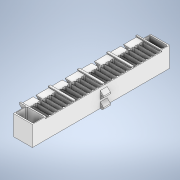
# Autodesk Inventor part: cajas_V2
Saved by Autodesk Inventor 2020.3 (Build 243373000, 373)
## iProperties
Created: 2021-02-18
Part Number: cajas_V2
Material: PET Plastic
Document SubType Name: Modeling
Designer: juanp
Density: 1.541 g/cm^3
Appearance: Polycarbonate - Clear
Author: juanp
Autodesk Inventor part; units mm, degrees
ref_plane "YZ Plane" through (0, 0, 0) normal (1, 0, 0) x (0, 1, 0)
ref_plane "XZ Plane" through (0, 0, 0) normal (0, 1, 0) x (-1, 0, 0)
ref_plane "XY Plane" through (0, 0, 0) normal (0, 0, 1) x (1, 0, 0)
sketch "Sketch1" plane through (0, 0, 0) normal (0, 1, 0) x (-1, 0, 0)
  line L0 (0, 0) -> (54, 0) construction
  line L1 (54, 0) -> (54, -330)
  line L2 (0, -330) -> (0, 0)
  line L3 (52, -4) -> (2, -4) construction
  line L4 (2, -4) -> (2, -15.1667)
  line L5 (2, -15.1667) -> (52, -15.1667)
  line L6 (52, -15.1667) -> (52, -4)
  line L7 (52, -19.1667) -> (2, -19.1667)
  line L8 (2, -19.1667) -> (2, -30.3333)
  line L9 (2, -30.3333) -> (52, -30.3333)
  line L10 (52, -30.3333) -> (52, -19.1667)
  line L11 (52, -32.3333) -> (2, -32.3333)
  line L12 (2, -32.3333) -> (2, -43.5)
  line L13 (2, -43.5) -> (52, -43.5)
  line L14 (52, -43.5) -> (52, -32.3333)
  line L15 (52, -45.5) -> (2, -45.5)
  line L16 (2, -45.5) -> (2, -56.6667)
  line L17 (2, -56.6667) -> (52, -56.6667)
  line L18 (52, -56.6667) -> (52, -45.5)
  line L19 (52, -58.6667) -> (2, -58.6667)
  line L20 (2, -58.6667) -> (2, -69.8333)
  line L21 (2, -69.8333) -> (52, -69.8333)
  line L22 (52, -69.8333) -> (52, -58.6667)
  line L23 (52, -71.8333) -> (2, -71.8333)
  line L24 (2, -71.8333) -> (2, -83)
  line L25 (2, -83) -> (52, -83)
  line L26 (52, -83) -> (52, -71.8333)
  line L27 (52, -85) -> (2, -85)
  line L28 (2, -85) -> (2, -96.1667)
  line L29 (2, -96.1667) -> (52, -96.1667)
  line L30 (52, -96.1667) -> (52, -85)
  line L31 (52, -102.1667) -> (2, -102.1667)
  line L32 (2, -102.1667) -> (2, -113.3333)
  line L33 (2, -113.3333) -> (52, -113.3333)
  line L34 (52, -113.3333) -> (52, -102.1667)
  line L35 (52, -115.3333) -> (2, -115.3333)
  line L36 (2, -115.3333) -> (2, -126.5)
  line L37 (2, -126.5) -> (52, -126.5)
  line L38 (52, -126.5) -> (52, -115.3333)
  line L39 (52, -128.5) -> (2, -128.5)
  line L40 (2, -128.5) -> (2, -139.6667)
  line L41 (2, -139.6667) -> (52, -139.6667)
  line L42 (52, -139.6667) -> (52, -128.5)
  line L43 (52, -141.6667) -> (2, -141.6667)
  line L44 (2, -141.6667) -> (2, -152.8333)
  line L45 (2, -152.8333) -> (52, -152.8333)
  line L46 (52, -152.8333) -> (52, -141.6667)
  line L47 (52, -154.8333) -> (2, -154.8333)
  line L48 (2, -154.8333) -> (2, -166)
  line L49 (2, -166) -> (52, -166)
  line L50 (52, -166) -> (52, -154.8333)
  line L51 (52, -168) -> (2, -168)
  line L52 (2, -168) -> (2, -179.1667)
  line L53 (2, -179.1667) -> (52, -179.1667)
  line L54 (52, -179.1667) -> (52, -168)
  line L55 (52, -185.1667) -> (2, -185.1667)
  line L56 (2, -185.1667) -> (2, -196.3333)
  line L57 (2, -196.3333) -> (52, -196.3333)
  line L58 (52, -196.3333) -> (52, -185.1667)
  line L59 (52, -198.3333) -> (2, -198.3333)
  line L60 (2, -198.3333) -> (2, -209.5)
  line L61 (2, -209.5) -> (52, -209.5)
  line L62 (52, -209.5) -> (52, -198.3333)
  line L63 (52, -211.5) -> (2, -211.5)
  line L64 (2, -211.5) -> (2, -222.6667)
  line L65 (2, -222.6667) -> (52, -222.6667)
  line L66 (52, -222.6667) -> (52, -211.5)
  line L67 (52, -224.6667) -> (2, -224.6667)
  line L68 (2, -224.6667) -> (2, -235.8333)
  line L69 (2, -235.8333) -> (52, -235.8333)
  line L70 (52, -235.8333) -> (52, -224.6667)
  line L71 (54, -330) -> (54, -349.1667)
  line L72 (54, -349.1667) -> (0, -349.1667) construction
  line L73 (0, -349.1667) -> (0, -330)
  line L74 (52, -237.8333) -> (2, -237.8333)
  line L75 (2, -237.8333) -> (2, -249)
  line L76 (2, -249) -> (52, -249)
  line L77 (52, -249) -> (52, -237.8333)
  line L78 (52, -251) -> (2, -251)
  line L79 (2, -251) -> (2, -262.1667)
  line L80 (2, -262.1667) -> (52, -262.1667)
  line L81 (52, -262.1667) -> (52, -251)
  line L82 (52, -268.1667) -> (2, -268.1667)
  line L83 (2, -268.1667) -> (2, -279.3333)
  line L84 (2, -279.3333) -> (52, -279.3333)
  line L85 (52, -279.3333) -> (52, -268.1667)
  line L86 (52, -281.3333) -> (2, -281.3333)
  line L87 (2, -281.3333) -> (2, -292.5)
  line L88 (2, -292.5) -> (52, -292.5)
  line L89 (52, -292.5) -> (52, -281.3333)
  line L90 (52, -294.5) -> (2, -294.5)
  line L91 (2, -294.5) -> (2, -305.6667)
  line L92 (2, -305.6667) -> (52, -305.6667)
  line L93 (52, -305.6667) -> (52, -294.5)
  line L94 (52, -307.6667) -> (2, -307.6667)
  line L95 (2, -307.6667) -> (2, -318.8333)
  line L96 (2, -318.8333) -> (52, -318.8333)
  line L97 (52, -318.8333) -> (52, -307.6667)
  line L98 (52, -320.8333) -> (2, -320.8333)
  line L99 (2, -320.8333) -> (2, -332)
  line L100 (2, -332) -> (52, -332)
  line L101 (52, -332) -> (52, -320.8333)
  line L102 (52, -334) -> (2, -334)
  line L103 (2, -334) -> (2, -345.1667)
  line L104 (2, -345.1667) -> (52, -345.1667)
  line L105 (52, -345.1667) -> (52, -334)
  line L106 (52, -4) -> (52, 16.4167)
  line L107 (52, 16.4167) -> (2, 16.4167)
  line L108 (2, 16.4167) -> (2, -4)
  line L109 (54, 0) -> (54, 20.4167)
  line L110 (54, 20.4167) -> (0, 20.4167)
  line L111 (0, 20.4167) -> (0, 0)
  line L112 (0, -349.1667) -> (0, -369.5833)
  line L113 (0, -369.5833) -> (54, -369.5833)
  line L114 (54, -369.5833) -> (54, -349.1667)
  line L115 (52, -339.5833) -> (104.9487, -339.5833) construction
  line L116 (104.9487, -339.5833) -> (104.9487, -9.5833) construction
  line L117 (104.9487, -9.5833) -> (52, -9.5833) construction
  line L118 (2, -349.1667) -> (52, -349.1667)
  line L119 (52, -349.1667) -> (52, -365.5833)
  line L120 (52, -365.5833) -> (2, -365.5833)
  line L121 (2, -365.5833) -> (2, -349.1667)
  point P0 (104.9487, -174.5833)
  dimension "d2" = 2
  dimension "d3" = 4
  dimension "d4" = 2
  dimension "d5" = 50
  dimension "d6" = 4
  dimension "d7" = 2
  dimension "d8" = 2
  dimension "d9" = 2
  dimension "d10" = 2
  dimension "d11" = 2
  dimension "d12" = 6
  dimension "d13" = 2
  dimension "d14" = 2
  dimension "d15" = 2
  dimension "d16" = 2
  dimension "d17" = 2
  dimension "d18" = 6
  dimension "d19" = 2
  dimension "d20" = 2
  dimension "d21" = 2
  dimension "d24" = 11.1667
  dimension "d35" = 2
  dimension "d36" = 2
  dimension "d37" = 6
  dimension "d38" = 2
  dimension "d39" = 2
  dimension "d40" = 2
  dimension "d41" = 2
  dimension "d42" = 2
  dimension "d59" = 4
  dimension "d60" = 330
  dimension "d212" = 4
  dimension "d332" = 195
  dimension "d333" = 195
  dimension "d334" = 4
  constraints: 244 end point, 53 parallel, 37 perpendicular, 34 equal length, 33 point on line, 28 horizontal, 8 collinear, 5 vertical, 3 midpoint
  measures "d2" distance between parallel lines of L1 L6
  measures "d3" distance between parallel lines of L0 L3
  measures "d4" distance between parallel lines of L4 L2
  measures "d5" distance of L3.start L3.end
  measures "d6" distance between parallel lines of L7 L5
  measures "d7" distance between parallel lines of L11 L9
  measures "d8" distance between parallel lines of L15 L13
  measures "d9" distance between parallel lines of L19 L17
  measures "d10" distance between parallel lines of L21 L23
  measures "d11" distance between parallel lines of L27 L25
  measures "d12" distance between parallel lines of L31 L29
  measures "d13" distance between parallel lines of L35 L33
  measures "d14" distance between parallel lines of L39 L37
  measures "d15" distance between parallel lines of L43 L41
  measures "d16" distance between parallel lines of L47 L45
  measures "d17" distance between parallel lines of L51 L49
  measures "d18" distance between parallel lines of L55 L53
  measures "d19" distance between parallel lines of L59 L57
  measures "d20" distance between parallel lines of L63 L61
  measures "d21" distance between parallel lines of L67 L65
  measures "d24" distance of L61.end L59.start
  measures "d35" distance between parallel lines of L69 L74
  measures "d36" distance between parallel lines of L78 L76
  measures "d37" distance between parallel lines of L82 L80
  measures "d38" distance between parallel lines of L86 L84
  measures "d39" distance between parallel lines of L90 L88
  measures "d40" distance between parallel lines of L94 L92
  measures "d41" distance between parallel lines of L98 L96
  measures "d42" distance between parallel lines of L102 L100
  measures "d59" distance between parallel lines of L72 L104
  measures "d60" distance of L117.end L115.start
  measures "d212" distance between parallel lines of L107 L110
  measures "d332" distance from line of L110 point (104.949, -174.583)
  measures "d333" distance from line of L113 point (104.949, -174.583)
  measures "d334" distance between parallel lines of L113 L120
extrude "Extrusion1" add sketch "Sketch1" along normal blind 50
sketch "Sketch3" plane through (0, 0, 0) normal (0, -1, 0) x (1, 0, 0)
  line L0 (-54, -369.5833) -> (-54, 20.4167) projected
  line L1 (0, 20.4167) -> (0, -369.5833) projected
  line L2 (-54, 20.4167) -> (0, 20.4167) projected
  line L3 (0, -369.5833) -> (-54, -369.5833) projected
extrude "Extrusion3" add sketch "Sketch3" along normal blind 2
chamfer "Chamfer4" distance 2 angle 45 208 edges at (-52, 25, -128.5) (-2, 25, -126.5) (-52, 25, -141.6667) (-52, 25, -179.1667) (-52, 25, -185.1667) (-2, 25, -141.6667) (-2, 25, -139.6667) (-52, 25, -115.3333) (-2, 25, -115.3333) (-2, 25, -345.1667) (-52, 25, -345.1667) (-2, 25, -128.5) (-2, 25, -332) (-2, 25, -334) (-52, 25, -334) (-52, 25, -332) (-2, 25, -320.8333) (-52, 25, -318.8333) (-2, 25, -318.8333) (-52, 25, -320.8333) (-2, 25, -307.6667) (-52, 25, -305.6667) (-52, 25, -307.6667) (-2, 25, -305.6667) (-2, 25, -294.5) (-52, 25, -292.5) (-2, 25, -292.5) (-52, 25, -294.5) (-2, 25, -281.3333) (-2, 25, -268.1667) (-52, 25, -279.3333) (-2, 25, -279.3333) (-52, 25, -281.3333) (-2, 25, -166) (-2, 25, -168) (-2, 25, -179.1667) (-2, 25, -196.3333) (-2, 25, -185.1667) (-2, 25, -209.5) (-2, 25, -198.3333) (-52, 0, -173.5833) (-2, 0, -173.5833) (-27, 0, -179.1667) (-27, 0, -185.1667) (-52, 0, -190.75) (-2, 0, -190.75) (-2, 0, -203.9167) (-27, 0, -198.3333) (-52, 0, -203.9167) (-27, 0, -196.3333) (-52, 0, -217.0833) (-2, 0, -217.0833) (-27, 0, -222.6667) (-27, 0, -209.5) (-52, 25, -196.3333) (-52, 25, -198.3333) (-52, 25, -209.5) (-2, 25, -211.5) (-52, 25, -211.5) (-52, 25, -222.6667) (-2, 25, -222.6667) (-2, 25, -224.6667) (-52, 25, -224.6667) (-2, 25, -251) (-52, 25, -249) (-2, 25, -249) (-52, 25, -251) (-2, 25, -262.1667) (-52, 25, -262.1667) (-52, 25, -268.1667) (-27, 0, -211.5) (-27, 0, -224.6667) (-52, 0, -230.25) (-2, 0, -230.25) (-27, 0, -235.8333) (-27, 0, -237.8333) (-52, 0, -243.4167) (-2, 0, -243.4167) (-27, 0, -249) (-27, 0, -251) (-52, 0, -256.5833) (-27, 0, -262.1667) (-27, 0, -268.1667) (-52, 0, -273.75) (-27, 0, -279.3333) (-2, 0, -273.75) (-52, 0, -286.9167) (-27, 0, -292.5) (-2, 0, -256.5833) (-27, 0, -281.3333) (-2, 0, -286.9167) (-27, 0, -294.5) (-52, 0, -300.0833) (-2, 0, -300.0833) (-27, 0, -305.6667) (-27, 0, -307.6667) (-52, 0, -313.25) (-2, 0, -313.25) (-27, 0, -318.8333) (-27, 0, -320.8333) (-27, 0, -332) (-2, 0, -326.4167) (-27, 0, -334) (-2, 0, -339.5833) (-27, 0, -345.1667) (-52, 0, -339.5833) (-52, 0, -326.4167) (-2, 25, -237.8333) (-2, 25, -235.8333) (-52, 25, -235.8333) (-52, 25, -237.8333) (-52, 25, -126.5) (-52, 25, -113.3333) (-2, 25, -113.3333) (-2, 25, -102.1667) (-52, 25, -102.1667) (-52, 25, -96.1667) (-2, 25, -96.1667) (-2, 25, -85) (-52, 25, -85) (-27, 0, -96.1667) (-2, 0, -90.5833) (-27, 0, -85) (-27, 0, -83) (-2, 0, -77.4167) (-27, 0, -71.8333) (-52, 0, -77.4167) (-52, 0, -90.5833) (-52, 25, -83) (-2, 25, -83) (-2, 25, -71.8333) (-52, 25, -71.8333) (-52, 25, -69.8333) (-2, 25, -69.8333) (-2, 25, -58.6667) (-52, 25, -58.6667) (-52, 25, -56.6667) (-52, 25, -45.5) (-52, 25, -43.5) (-2, 25, -56.6667) (-52, 25, -32.3333) (-2, 25, -43.5) (-52, 25, -30.3333) (-2, 25, -32.3333) (-2, 25, -30.3333) (-52, 25, -19.1667) (-2, 25, -19.1667) (-2, 25, -45.5) (-52, 0, -24.75) (-52, 25, -15.1667) (-2, 25, -15.1667) (-27, 0, -43.5) (-27, 0, -32.3333) (-2, 0, -37.9167) (-27, 0, -30.3333) (-2, 0, -24.75) (-27, 0, -19.1667) (-52, 0, -37.9167) (-27, 0, -69.8333) (-52, 0, -64.25) (-2, 0, -64.25) (-27, 0, -58.6667) (-27, 0, -56.6667) (-2, 0, -51.0833) (-27, 0, -45.5) (-52, 0, -51.0833) (-2, 25, -154.8333) (-2, 25, -152.8333) (-52, 25, -152.8333) (-52, 25, -139.6667) (-27, 0, -168) (-27, 0, -166) (-27, 0, -154.8333) (-2, 0, -160.4167) (-27, 0, -152.8333) (-2, 0, -147.25) (-27, 0, -141.6667) (-2, 0, -134.0833) (-27, 0, -128.5) (-52, 0, -147.25) (-52, 0, -160.4167) (-27, 0, -102.1667) (-52, 0, -107.75) (-2, 0, -107.75) (-27, 0, -113.3333) (-27, 0, -115.3333) (-27, 0, -126.5) (-2, 0, -120.9167) (-27, 0, -139.6667) (-52, 0, -134.0833) (-52, 0, -120.9167) (-52, 25, -154.8333) (-52, 25, -166) (-52, 25, -168) (-2, 25, 16.4167) (-52, 25, 16.4167) (-27, 0, 16.4167) (-52, 0, 0.625) (-27, 0, -15.1667) (-2, 0, 0.625) (-27, 0, -365.5833) (-2, 0, -357.375) (-2, 25, -365.5833) (-52, 25, -349.1667) (-52, 0, -357.375) (-27, 0, -349.1667) (-2, 25, -349.1667) (-52, 25, -365.5833)
ref_plane "Plano medio efectivo" through (-4, 2, -174.5833) normal (0, 0, -1) x (-1, 0, 0)
sketch "Sketch57" plane through (-4, 50, -349.1667) normal (0, 0, -1) x (-1, 0, 0)
  line L0 (50, -52) -> (50, 0) projected
  line L1 (50, 0) -> (67.933, 0)
  line L2 (67.933, 0) -> (50, -17.933)
  point P0 (-4, -50)
  dimension "d335" = 45
  dimension "d336" = 17.933
  constraints: 4 end point, 1 horizontal, 1 point on line
  measures "d335" angle of L0 L2
  measures "d336" distance of L0.end L1.end
extrude "Extrusion46" add sketch "Sketch57" against normal up to surface (334 mm away)
sketch "Sketch58" plane through (0, 50, 0) normal (0, 1, 0) x (1, 0, 0)
  line L0 (0, -20.4167) -> (0, 369.5833) projected
  line L1 (-71.933, 349.1667) -> (-71.933, 15.1667) projected
  line L2 (-71.933, 349.1667) -> (-54, 349.1667) projected
  line L3 (-71.933, 349.1667) -> (0, 349.1667)
  line L4 (-71.933, 15.1667) -> (0, 15.1667)
  line L5 (-4, 19.1667) -> (-50, 19.1667) projected
  line L6 (-27, 19.1667) -> (-27, 15.1667) construction
  line L7 (-50, 15.1667) -> (-4, 15.1667) projected
  line L8 (-4, 102.1667) -> (-50, 102.1667) projected
  line L9 (-27, 102.1667) -> (-27, 100.1667) construction
  line L10 (-27, 100.1667) -> (-27, 98.1667) construction
  line L11 (-27, 98.1667) -> (-27, 96.1667) construction
  line L12 (-4, 96.1667) -> (-50, 96.1667) projected
  line L13 (-4, 179.1667) -> (-50, 179.1667) projected
  line L14 (-27, 179.1667) -> (-27, 181.1667) construction
  line L15 (-27, 181.1667) -> (-27, 183.1667) construction
  line L16 (-27, 183.1667) -> (-27, 185.1667) construction
  line L17 (-4, 185.1667) -> (-50, 185.1667) projected
  line L18 (-50, 262.1667) -> (-4, 262.1667) projected
  line L19 (-27, 262.1667) -> (-27, 264.1667) construction
  line L20 (-27, 264.1667) -> (-27, 266.1667) construction
  line L21 (-27, 266.1667) -> (-27, 268.1667) construction
  line L22 (-4, 268.1667) -> (-50, 268.1667) projected
  line L23 (-4, 345.1667) -> (-50, 345.1667) projected
  line L24 (-4, 349.1667) -> (-50, 349.1667) projected
  line L25 (-27, 349.1667) -> (-27, 345.1667) construction
  line L26 (0, 347.1667) -> (-71.933, 347.1667)
  line L27 (-71.933, 266.1667) -> (0, 266.1667)
  line L28 (-71.933, 264.1667) -> (0, 264.1667)
  line L29 (0, 183.1667) -> (-71.933, 183.1667)
  line L30 (-71.933, 181.1667) -> (0, 181.1667)
  line L31 (-71.933, 98.1667) -> (0, 98.1667)
  line L32 (0, 100.1667) -> (-71.933, 100.1667)
  line L33 (0, 17.1667) -> (-71.933, 17.1667)
  point P0 (-27, 347.1667)
  point P1 (-27, 17.1667)
  constraints: 42 end point, 12 midpoint, 12 point on line, 6 collinear, 6 horizontal, 4 parallel, 2 vertical, 20 other
extrude "Extrusion47" add sketch "Sketch58" along normal blind 3 contours L4 L1 L33 L0 | L31 L1 L32 L0 | L30 L1 L29 L0 | L28 L1 L27 L0 | L26 L1 L2 L3 L0
sketch "Sketch59" plane through (0, 53, 0) normal (0, 1, 0) x (1, 0, 0)
  line L0 (0, 266.1667) -> (-71.933, 266.1667) projected
  line L1 (-71.933, 266.1667) -> (-71.933, 264.1667) projected
  line L2 (-71.933, 264.1667) -> (0, 264.1667) projected
  line L3 (0, 183.1667) -> (-71.933, 183.1667) projected
  line L4 (-71.933, 183.1667) -> (-71.933, 181.1667) projected
  line L5 (-71.933, 181.1667) -> (0, 181.1667) projected
  line L6 (0, 100.1667) -> (-71.933, 100.1667) projected
  line L7 (-71.933, 100.1667) -> (-71.933, 98.1667) projected
  line L8 (-71.933, 98.1667) -> (0, 98.1667) projected
  line L9 (0, 17.1667) -> (-71.933, 17.1667) projected
  line L10 (-71.933, 17.1667) -> (-71.933, 15.1667) projected
  line L11 (-71.933, 15.1667) -> (0, 15.1667) projected
  line L12 (0, 98.1667) -> (0, 100.1667) projected
  line L13 (0, 349.1667) -> (-71.933, 349.1667) projected
  line L14 (-71.933, 349.1667) -> (-71.933, 347.1667) projected
  line L15 (-71.933, 347.1667) -> (0, 347.1667) projected
  line L16 (-71.933, 98.1667) -> (-71.933, 17.1667) projected
  line L17 (-71.933, 181.1667) -> (-71.933, 100.1667) projected
  line L18 (-71.933, 264.1667) -> (-71.933, 183.1667) projected
  line L19 (-71.933, 347.1667) -> (-71.933, 266.1667) projected
  line L20 (-71.933, 345.1667) -> (0, 345.1667)
  line L21 (0, 345.1667) -> (0, 268.1667)
  line L22 (0, 268.1667) -> (-71.933, 268.1667)
  line L23 (-71.933, 268.1667) -> (-71.933, 345.1667)
  line L24 (-71.933, 262.1667) -> (0, 262.1667)
  line L25 (0, 262.1667) -> (0, 185.1667)
  line L26 (0, 185.1667) -> (-71.933, 185.1667)
  line L27 (-71.933, 185.1667) -> (-71.933, 262.1667)
  line L28 (-71.933, 179.1667) -> (0, 179.1667)
  line L29 (0, 179.1667) -> (0, 102.1667)
  line L30 (0, 102.1667) -> (-71.933, 102.1667)
  line L31 (-71.933, 102.1667) -> (-71.933, 179.1667)
  line L32 (-71.933, 96.1667) -> (0, 96.1667)
  line L33 (0, 96.1667) -> (0, 19.1667)
  line L34 (0, 19.1667) -> (-71.933, 19.1667)
  line L35 (-71.933, 19.1667) -> (-71.933, 96.1667)
  line L36 (0, 181.1667) -> (0, 183.1667) projected
  line L37 (0, 15.1667) -> (0, 17.1667) projected
  line L38 (0, 264.1667) -> (0, 266.1667) projected
  line L39 (0, 347.1667) -> (0, 349.1667) projected
  line L40 (0, 183.1667) -> (0, 264.1667) projected
  line L41 (0, 100.1667) -> (0, 181.1667) projected
  line L42 (0, 266.1667) -> (0, 347.1667) projected
  line L43 (0, 17.1667) -> (0, 98.1667) projected
  point P0 (0, 0)
  point P1 (-71.933, 268.1667)
  point P2 (-71.933, 185.1667)
  point P3 (-71.933, 102.1667)
  point P4 (-71.933, 19.1667)
  point P5 (0, 345.1667)
  point P6 (0, 262.1667)
  point P7 (0, 179.1667)
  dimension "d341" = 2
  dimension "d343" = 2
  dimension "d344" = 2
  dimension "d345" = 2
  dimension "d346" = 2
  dimension "d347" = 2
  dimension "d348" = 2
  dimension "d349" = 2
  constraints: 32 end point, 8 parallel, 5 point on line, 4 horizontal, 4 perpendicular, 3 collinear
  measures "d341" distance between parallel lines of L15 L20
  measures "d343" distance between parallel lines of L0 L22
  measures "d344" distance between parallel lines of L24 L2
  measures "d345" distance between parallel lines of L3 L26
  measures "d346" distance between parallel lines of L28 L5
  measures "d347" distance between parallel lines of L6 L30
  measures "d348" distance between parallel lines of L32 L8
  measures "d349" distance between parallel lines of L9 L34
extrude "Extrusion48" add sketch "Sketch59" along normal blind 2 contours L38 L2 L1 L0 | L0 L19 L22 L42 | L40 L24 L18 L2 | L20 L19 L15 L42 | L40 L3 L18 L26 | L15 L14 L13 L39 | L36 L5 L4 L3 | L41 L28 L17 L5 | L41 L6 L17 L30 | L12 L8 L7 L6 | L43 L32 L16 L8 | L43 L9 L16 L34 | L37 L11 L10 L9
chamfer "Chamfer11" distance 1.999 angle 45 8 edges at (-35.9665, 53, -17.1667) (-35.9665, 53, -98.1667) (-35.9665, 53, -100.1667) (-35.9665, 53, -181.1667) (-35.9665, 53, -183.1667) (-35.9665, 53, -264.1667) (-35.9665, 53, -266.1667) (-35.9665, 53, -347.1667)
sketch "Sketch60" plane through (0, 50, 0) normal (0, 1, 0) x (1, 0, 0)
  line L0 (-50, 15.1667) -> (-54, 15.1667) projected
  line L1 (-54, 15.1667) -> (-54, -20.4167) projected
  line L2 (-54, -20.4167) -> (0, -20.4167) projected
  line L3 (0, -20.4167) -> (0, 15.1667) projected
  line L4 (0, 15.1667) -> (-4, 15.1667) projected
  line L5 (-2, 13.1667) -> (-4, 15.1667) projected
  line L6 (-2, 13.1667) -> (-2, -14.4167) projected
  line L7 (-4, -16.4167) -> (-2, -14.4167) projected
  line L8 (-4, -16.4167) -> (-50, -16.4167) projected
  line L9 (-52, -14.4167) -> (-50, -16.4167) projected
  line L10 (-52, -14.4167) -> (-52, 13.1667) projected
  line L11 (-50, 15.1667) -> (-52, 13.1667) projected
  line L12 (-4, 349.1667) -> (0, 349.1667) projected
  line L13 (0, 349.1667) -> (0, 369.5833) projected
  line L14 (0, 369.5833) -> (-54, 369.5833) projected
  line L15 (-54, 369.5833) -> (-54, 349.1667) projected
  line L16 (-54, 349.1667) -> (-50, 349.1667) projected
  line L17 (-52, 351.1667) -> (-50, 349.1667) projected
  line L18 (-52, 351.1667) -> (-52, 363.5833) projected
  line L19 (-50, 365.5833) -> (-52, 363.5833) projected
  line L20 (-50, 365.5833) -> (-4, 365.5833) projected
  line L21 (-2, 363.5833) -> (-4, 365.5833) projected
  line L22 (-2, 363.5833) -> (-2, 351.1667) projected
  line L23 (-4, 349.1667) -> (-2, 351.1667) projected
  point P0 (0, 0)
extrude "Extrusion49" add sketch "Sketch60" along normal up to surface (5 mm away)
sketch "Sketch61" plane through (0, 50, 0) normal (0, 1, 0) x (1, 0, 0)
  line L0 (-54, -20.4167) -> (-54, 369.5833) projected
  line L1 (-54, 15.1667) -> (-54, 349.1667) projected
  line L2 (-71.933, 347.1667) -> (-71.933, 266.1667) projected
  line L3 (-54, 310.4167) -> (-71.933, 310.4167)
  line L4 (-71.933, 310.4167) -> (-71.933, 302.9167)
  line L5 (-71.933, 302.9167) -> (-54, 302.9167)
  line L6 (-54, 302.9167) -> (-54, 310.4167)
  line L7 (-54, 227.4167) -> (-71.933, 227.4167)
  line L8 (-71.933, 227.4167) -> (-71.933, 219.9167)
  line L9 (-71.933, 219.9167) -> (-54, 219.9167)
  line L10 (-54, 219.9167) -> (-54, 227.4167)
  line L11 (-54, 144.4167) -> (-71.933, 144.4167)
  line L12 (-71.933, 144.4167) -> (-71.933, 136.9167)
  line L13 (-71.933, 136.9167) -> (-54, 136.9167)
  line L14 (-54, 136.9167) -> (-54, 144.4167)
  line L15 (-54, 61.4167) -> (-71.933, 61.4167)
  line L16 (-71.933, 61.4167) -> (-71.933, 53.9167)
  line L17 (-71.933, 53.9167) -> (-54, 53.9167)
  line L18 (-54, 53.9167) -> (-54, 61.4167)
  point P0 (0, 0)
  point P1 (-71.933, 306.6667)
  point P2 (-71.933, 223.6667)
  point P3 (-71.933, 140.6667)
  point P4 (-71.933, 57.6667)
  point P5 (-54, 144.4167)
  dimension "d359" = 7.5
  dimension "d362" = 83
  constraints: 32 end point, 2 midpoint, 2 parallel, 2 point on line, 1 horizontal, 1 perpendicular, 1 vertical, 27 other
  measures "d359" distance between parallel lines of L5 L3
  measures "d362" distance of L3.start L7.start
extrude "Extrusion50" cut sketch "Sketch61" against normal up to next
ref_plane "Work Plane14" through (-54, 50, -297.5167) normal (0, 0, -1) x (-1, 0, 0)
sketch "Sketch62" plane through (-54, 50, -297.5167) normal (0, 0, -1) x (-1, 0, 0)
  line L0 (0, -17.933) -> (17.933, 0) projected
  line L1 (0, -52) -> (0, 5) projected
  line L2 (0, -50.233) -> (10, -40.233)
  line L3 (0, -50.233) -> (14.1421, -50.233) construction
  line L4 (10, -40.233) -> (10, -7.933)
  line L5 (10, -40.233) -> (0, -40.233) construction
  line L6 (5, -40.233) -> (5, -34.183) construction
  line L7 (5, -34.183) -> (5, -19.183) construction
  circle A0 centre (5, -34.183) radius 1.65
  circle A1 centre (5, -19.183) radius 1.65
  point P0 (-54, -50)
  dimension "d387" = 45
  dimension "d388" = 6.05
  dimension "d389" = 15
  dimension "d390" = 5
  dimension "d391" = 11.767
  dimension "d392" = 3.3
  constraints: 12 end point, 4 point on line, 2 centre point, 2 coincident, 2 horizontal, 2 vertical, 1 equal length, 1 equal radius, 1 midpoint
  measures "d387" angle of L3 L2
  measures "d388" distance of L6.start L6.end
  measures "d389" distance of L6.end L7.end
  measures "d390" distance between parallel lines of L1 L6
  measures "d391" distance from line of L5 L1.start
  measures "d392" diameter of A0
extrude "Extrusion51" add sketch "Sketch62" against normal blind 5
sketch "Sketch63" plane through (-54, 50, -297.5167) normal (0, 0, -1) x (-1, 0, 0)
  circle A0 centre (5, -19.183) radius 1.65 projected
  line L0 (3.4123, -16.433) -> (6.5877, -16.433)
  line L1 (6.5877, -16.433) -> (8.1754, -19.183)
  line L2 (8.1754, -19.183) -> (6.5877, -21.933)
  line L3 (6.5877, -21.933) -> (3.4123, -21.933)
  line L4 (3.4123, -21.933) -> (1.8246, -19.183)
  line L5 (1.8246, -19.183) -> (3.4123, -16.433)
  circle A1 centre (5, -34.183) radius 1.65 projected
  line L6 (3.4123, -31.433) -> (6.5877, -31.433)
  line L7 (6.5877, -31.433) -> (8.1754, -34.183)
  line L8 (8.1754, -34.183) -> (6.5877, -36.933)
  line L9 (6.5877, -36.933) -> (3.4123, -36.933)
  line L10 (3.4123, -36.933) -> (1.8246, -34.183)
  line L11 (1.8246, -34.183) -> (3.4123, -31.433)
  point P0 (-54, -50)
  dimension "d398" = 5.5
  constraints: 24 end point, 2 coincident, 2 horizontal, 1 parallel, 26 other
  measures "d398" distance between parallel lines of L0 L3
extrude "Extrusion52" cut sketch "Sketch63" against normal blind 2.5
pattern_linear "Rectangular Pattern9" count 4 spacing 83 along (0, 0, 1) of "Extrusion51", "Extrusion52"
ref_plane "Plano de corte" through (-4, 50, -182.1667) normal (0, 0, -1) x (-1, 0, 0)
sketch "Sketch65" plane through (-4, 50, -182.1667) normal (0, 0, -1) x (-1, 0, 0)
  line L0 (-13.3, -45.4239) -> (-10.5761, -42.7)
  line L1 (-10.5761, -42.7) -> (-6.7239, -42.7) construction
  line L2 (-6.7239, -42.7) -> (-4, -45.4239) construction
  line L3 (-4, -45.4239) -> (-4, -49.2761) construction
  line L4 (-4, -49.2761) -> (-6.7239, -52) construction
  line L5 (-6.7239, -52) -> (-10.5761, -52)
  line L6 (-10.5761, -52) -> (-13.3, -49.2761)
  line L7 (-13.3, -49.2761) -> (-13.3, -45.4239)
  line L8 (-4, -17.2569) -> (-4, -21.1091) construction
  line L9 (-4, -21.1091) -> (-6.7239, -23.833) construction
  line L10 (-6.7239, -23.833) -> (-10.5761, -23.833) construction
  line L11 (-10.5761, -23.833) -> (-13.3, -21.1091)
  line L12 (-13.3, -21.1091) -> (-13.3, -17.2569)
  line L13 (-13.3, -17.2569) -> (-10.5761, -14.533)
  line L14 (-10.5761, -14.533) -> (-6.7239, -14.533) construction
  line L15 (-6.7239, -14.533) -> (-4, -17.2569) construction
  line L16 (50.35, -17.2569) -> (53.0739, -14.533) construction
  line L17 (53.0739, -14.533) -> (56.9261, -14.533) construction
  line L18 (56.9261, -14.533) -> (59.65, -17.2569)
  line L19 (59.65, -17.2569) -> (59.65, -21.1091)
  line L20 (59.65, -21.1091) -> (56.9261, -23.833)
  line L21 (56.9261, -23.833) -> (53.0739, -23.833) construction
  line L22 (53.0739, -23.833) -> (50.35, -21.1091) construction
  line L23 (50.35, -21.1091) -> (50.35, -17.2569) construction
  line L24 (59.65, -49.2761) -> (56.9261, -52)
  line L25 (56.9261, -52) -> (53.0739, -52)
  line L26 (53.0739, -52) -> (50.35, -49.2761) construction
  line L27 (50.35, -49.2761) -> (50.35, -45.4239) construction
  line L28 (50.35, -45.4239) -> (53.0739, -42.7) construction
  line L29 (53.0739, -42.7) -> (56.9261, -42.7) construction
  line L30 (56.9261, -42.7) -> (59.65, -45.4239)
  line L31 (59.65, -45.4239) -> (59.65, -49.2761)
  line L32 (-8.65, -19.183) -> (55, -19.183) construction
  line L33 (55, -19.183) -> (55, -47.35) construction
  line L34 (55, -47.35) -> (-8.65, -47.35) construction
  line L35 (-8.65, -47.35) -> (-8.65, -19.183) construction
  line L36 (-8.65, -19.183) -> (55, -47.35) construction
  line L37 (55, -19.183) -> (-8.65, -47.35) construction
  circle A0 centre (-8.65, -19.183) radius 1.65
  circle A1 centre (-8.65, -47.35) radius 1.65
  circle A2 centre (55, -47.35) radius 1.65
  circle A3 centre (55, -19.183) radius 1.65
  line L38 (-4, -52) -> (50, -52) projected
  circle A4 centre (55, -19.183) radius 1.65 projected
  line L39 (-4, 5) -> (-4, -52) projected
  line L40 (-10.5761, -14.533) -> (-4, -7.9569)
  line L41 (-10.5761, -23.833) -> (-4, -30.4091)
  line L42 (-10.5761, -42.7) -> (-4, -36.1239)
  line L43 (-6.7239, -52) -> (-4, -52)
  line L44 (50, -52) -> (53.0739, -52)
  line L45 (56.9261, -42.7) -> (50, -35.7739)
  line L46 (50, -50.233) -> (50, -17.933) projected
  line L47 (50, -30.7591) -> (56.9261, -23.833)
  line L48 (56.9261, -14.533) -> (55.163, -12.77)
  line L49 (50, -17.933) -> (67.933, 0) projected
  line L50 (50, -52) -> (50, 5) projected
  point P0 (23.175, -33.2665)
  dimension "d403" = 3
  constraints: 92 end point, 8 coincident, 8 collinear, 6 horizontal, 6 parallel, 6 point on line, 4 centre point, 4 equal radius, 2 midpoint, 1 concentric, 1 perpendicular, 68 other
  measures "d403" distance edge to line of A2 L31
extrude "Extrusion53" add sketch "Sketch65" along normal mid plane 20
sketch "Sketch66" plane through (-4, 50, -192.1667) normal (0, 0, -1) x (-1, 0, 0)
  circle A0 centre (-8.65, -19.183) radius 1.65 projected
  circle A1 centre (-8.65, -47.35) radius 1.65 projected
  circle A2 centre (55, -47.35) radius 1.65 projected
  circle A3 centre (55, -19.183) radius 1.65 projected
  line L0 (-7.0623, -21.933) -> (-10.2377, -21.933)
  line L1 (-10.2377, -21.933) -> (-11.8254, -19.183)
  line L2 (-11.8254, -19.183) -> (-10.2377, -16.433)
  line L3 (-10.2377, -16.433) -> (-7.0623, -16.433)
  line L4 (-7.0623, -16.433) -> (-5.4746, -19.183)
  line L5 (-5.4746, -19.183) -> (-7.0623, -21.933)
  line L6 (-11.8254, -47.35) -> (-10.2377, -44.6)
  line L7 (-10.2377, -44.6) -> (-7.0623, -44.6)
  line L8 (-7.0623, -44.6) -> (-5.4746, -47.35)
  line L9 (-5.4746, -47.35) -> (-7.0623, -50.1)
  line L10 (-7.0623, -50.1) -> (-10.2377, -50.1)
  line L11 (-10.2377, -50.1) -> (-11.8254, -47.35)
  line L12 (51.8246, -47.35) -> (53.4123, -44.6)
  line L13 (53.4123, -44.6) -> (56.5877, -44.6)
  line L14 (56.5877, -44.6) -> (58.1754, -47.35)
  line L15 (58.1754, -47.35) -> (56.5877, -50.1)
  line L16 (56.5877, -50.1) -> (53.4123, -50.1)
  line L17 (53.4123, -50.1) -> (51.8246, -47.35)
  circle A4 centre (55, -19.183) radius 1.65 projected
  line L18 (53.4123, -16.433) -> (56.5877, -16.433)
  line L19 (56.5877, -16.433) -> (58.1754, -19.183)
  line L20 (58.1754, -19.183) -> (56.5877, -21.933)
  line L21 (56.5877, -21.933) -> (53.4123, -21.933)
  line L22 (53.4123, -21.933) -> (51.8246, -19.183)
  line L23 (51.8246, -19.183) -> (53.4123, -16.433)
  point P0 (-4, -50)
  dimension "d406" = 5.5
  constraints: 48 end point, 4 coincident, 4 horizontal, 3 equal length, 52 other
  measures "d406" distance between parallel lines of L3 L0
extrude "Extrusion54" cut sketch "Sketch66" against normal blind 2.5
chamfer "Chamfer12" distance 0.6667 angle 45 48 edges at (-27, 50, -345.1667) (-27, 50, -334) (-27, 50, -332) (-27, 50, -320.8333) (-27, 50, -318.8333) (-27, 50, -307.6667) (-27, 50, -305.6667) (-27, 50, -294.5) (-27, 50, -292.5) (-27, 50, -281.3333) (-27, 50, -279.3333) (-27, 50, -262.1667) (-27, 50, -251) (-27, 50, -249) (-27, 50, -237.8333) (-27, 50, -235.8333) (-27, 50, -224.6667) (-27, 50, -222.6667) (-27, 50, -209.5) (-27, 50, -211.5) (-27, 50, -198.3333) (-27, 50, -196.3333) (-27, 50, -179.1667) (-27, 50, -168) (-27, 50, -166) (-27, 50, -154.8333) (-27, 50, -152.8333) (-27, 50, -141.6667) (-27, 50, -139.6667) (-27, 50, -128.5) (-27, 50, -126.5) (-27, 50, -115.3333) (-27, 50, -113.3333) (-27, 50, -96.1667) (-27, 50, -85) (-27, 50, -83) (-27, 50, -71.8333) (-27, 50, -69.8333) (-27, 50, -58.6667) (-27, 50, -56.6667) (-27, 50, -43.5) (-27, 50, -45.5) (-27, 50, -32.3333) (-27, 50, -30.3333) (-27, 50, -19.1667) (-27, 50, -102.1667) (-27, 50, -185.1667) (-27, 50, -268.1667)
equation "\"d2\" = grosor_pared"
equation "\"d5\" = largo_cajas"
equation "\"d7\" = grosor_pared"
equation "\"d8\" = grosor_pared"
equation "\"d10\" = grosor_pared"
equation "\"d14\" = grosor_pared"
equation "\"d15\" = grosor_pared"
equation "\"d16\" = grosor_pared"
equation "\"d19\" = grosor_pared"
equation "\"d20\" = grosor_pared"
equation "\"d21\" = grosor_pared"
equation "\"d25\" = altura_cajas"
equation "\"d32\" = grosor_pared"
equation "\"largo_cajas\" = 50"
equation "\"grosor_pared\" = 2"
equation "\"altura_cajas\" = 50"
body "Solid1"
